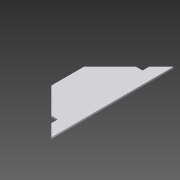
# Autodesk Inventor part: top long
Saved by Autodesk Inventor 2015 (Build 190159000, 159)
## iProperties
Created: 2019-04-10
Part Number: top long
Material: Generic
Document SubType Name: Modeling
Designer: Raptor
Density: 1 g/cm^3
Appearance: Snow
Author: Raptor
Autodesk Inventor part; units mm, degrees
ref_plane "YZ Plane" through (0, 0, 0) normal (1, 0, 0) x (0, 1, 0)
ref_plane "XZ Plane" through (0, 0, 0) normal (0, 1, 0) x (-1, 0, 0)
ref_plane "XY Plane" through (0, 0, 0) normal (0, 0, 1) x (1, 0, 0)
sketch "Sketch4" plane through (0, 0, 0) normal (0, 1, 0) x (-1, 0, 0)
  line L0 (0, 0) -> (0, -1500)
  line L1 (550, -950) -> (550, -550)
  line L2 (150, -150) -> (150, -230)
  line L3 (150, -230) -> (230, -230)
  line L4 (550, -550) -> (230, -230)
  line L5 (150, -150) -> (0, 0)
  line L6 (150, -1350) -> (150, -1270)
  line L7 (150, -1270) -> (230, -1270)
  line L8 (0, -1500) -> (150, -1350)
  line L9 (230, -1270) -> (550, -950)
  dimension "d8" = 1500
  dimension "d11" = 550
  dimension "d12" = 80
  dimension "d13" = 150
  dimension "d14" = 150
  dimension "d15" = 80
  dimension "d16" = 45
  constraints: 20 end point, 3 perpendicular, 3 vertical, 2 collinear, 1 parallel
  measures "d8" distance of L0.start L0.end
  measures "d11" distance between parallel lines of L0 L1
  measures "d12" distance of L2.start L2.end
  measures "d13" distance between parallel lines of L0 L2
  measures "d14" distance between parallel lines of L0 L6
  measures "d15" distance of L6.start L6.end
  measures "d16" angle of L0 L8
extrude "Extrusion1" add sketch "Sketch4" along normal blind 20
fillet "Fillet1" radius 5 1 edges at (-150, 10, -230)
fillet "Fillet2" radius 5 1 edges at (-150, 10, -1270)
body "Solid1"
